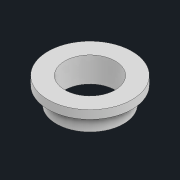
# Autodesk Inventor part: ProtectorBloqueo
Saved by Autodesk Inventor 2021 (Build 250183000, 183)
## iProperties
Created: 2021-05-07
Part Number: ProtectorBloqueo
Material: Generic
Document SubType Name: Modeling
Designer: GABRIEL LOL
Density: 1 g/cm^3
Appearance: Default
Author: GABRIEL LOL
Autodesk Inventor part; units mm, degrees
ref_plane "YZ Plane" through (0, 0, 0) normal (1, 0, 0) x (0, 1, 0)
ref_plane "XZ Plane" through (0, 0, 0) normal (0, 1, 0) x (-1, 0, 0)
ref_plane "XY Plane" through (0, 0, 0) normal (0, 0, 1) x (1, 0, 0)
sketch "Sketch1" plane through (0, 0, 0) normal (0, 0, 1) x (1, 0, 0)
  line L0 (0, 0) -> (1.5, 0) construction
  line L1 (1.5, 0) -> (1.5, 1.5)
  line L2 (1.5, 1.5) -> (2.5, 1.5)
  line L3 (2.5, 1.5) -> (2.5, 1)
  line L4 (1.5, 0) -> (2, 0)
  line L5 (2, 0) -> (2, 1)
  line L6 (2, 1) -> (2.5, 1)
  line L7 (0, -0.3) -> (0, 1.8) projected
  dimension "d0" = 1.5
  dimension "d1" = 1.5
  dimension "d2" = 1
  dimension "d3" = 0.5
  dimension "d4" = 0.5
  constraints: 14 end point, 3 horizontal, 3 perpendicular, 1 vertical
  measures "d0" distance of L0.start L0.end
  measures "d1" distance of L0.end L1.end
  measures "d2" distance of L1.end L2.end
  measures "d3" distance of L2.end L3.end
  measures "d4" distance of L0.end L4.end
revolve "Revolution1" add sketch "Sketch1" angle 360 about axis through (0, -10, 0) along (0, 1, 0)
body "Solid1"
